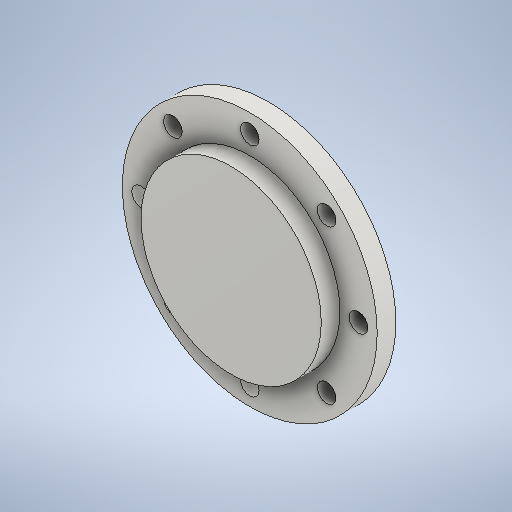
# Autodesk Inventor part: 07 CYLINDER FRONT COVER
Saved by Autodesk Inventor 2025.2 (Build 292293000, 293)
## iProperties
Created: 2025-05-29
Part Number: 07 CYLINDER FRONT COVER
Material: Steel AISI 1020 107 HR
Document SubType Name: Modeling
Designer: bless
Density: 7.87 g/cm^3
Appearance: Steel
Author: bless
Autodesk Inventor part; units mm, degrees
ref_plane "YZ Plane" through (0, 0, 0) normal (1, 0, 0) x (0, 1, 0)
ref_plane "XZ Plane" through (0, 0, 0) normal (0, 1, 0) x (-1, 0, 0)
ref_plane "XY Plane" through (0, 0, 0) normal (0, 0, 1) x (1, 0, 0)
sketch "Sketch1" plane through (0, 0, 0) normal (0, 0, 1) x (1, 0, 0)
  circle A0 centre (0, 0) radius 20.5
  dimension "d0" = 41
  constraints: 1 centre point, 1 coincident
  measures "d0" diameter of A0
extrude "Extrusion1" add sketch "Sketch1" along normal blind 3
sketch "Sketch2" plane through (0, 0, 3) normal (0, 0, 1) x (1, 0, 0)
  circle A0 centre (0, 0) radius 20.5 projected
  circle A1 centre (0, 0) radius 14.5
  dimension "d3" = 29
  constraints: 1 centre point, 1 coincident
  measures "d3" diameter of A1
extrude "Extrusion2" add sketch "Sketch2" along normal blind 3 contours A1
sketch "Sketch3" plane through (0, 0, 0) normal (0, 0, -1) x (-1, 0, 0)
  circle A0 centre (0, 0) radius 20.5 projected
  circle A1 centre (0, 0) radius 14.5
  dimension "d6" = 29
  constraints: 1 centre point, 1 coincident
  measures "d6" diameter of A1
extrude "Extrusion3" add sketch "Sketch3" along normal blind 2 contours A1
sketch "Sketch4" plane through (0, 0, 3) normal (0, 0, 1) x (1, 0, 0)
  circle A0 centre (0, 0) radius 14.5 projected
  circle A1 centre (0, 0) radius 20.5 projected
  circle A2 centre (0, 0) radius 17.5
  circle A3 centre (0, 17.5) radius 1.5
  circle A4 centre (-12.3744, 12.3744) radius 1.5
  circle A5 centre (-17.5, 0) radius 1.5
  circle A6 centre (-12.3744, -12.3744) radius 1.5
  circle A7 centre (0, -17.5) radius 1.5
  circle A8 centre (12.3744, -12.3744) radius 1.5
  circle A9 centre (17.5, 0) radius 1.5
  circle A10 centre (12.3744, 12.3744) radius 1.5
  dimension "d9" = 35
  dimension "d10" = 3
  dimension "d13" = 360
  constraints: 8 centre point, 2 vertical alignment, 1 coincident, 19 other
  measures "d10" diameter of A3
extrude "Extrusion4" cut sketch "Sketch4" against normal through all contours A2 A9 | A2 A9 | A10 A2 | A2 A10 | A8 A2 | A2 A8 | A3 A2 | A2 A3 | A7 A2 | A2 A7 | A4 A2 | A2 A4 | A6 A2 | A2 A6 | A5 A2 | A2 A5
body "Solid1"
